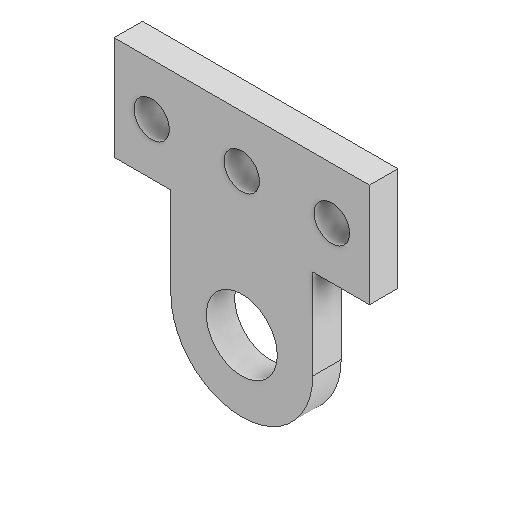
# Autodesk Inventor part: Suporte Coletor - Intake
Saved by Autodesk Inventor 2025.3 (Build 293356000, 356)
## iProperties
Created: 2026-05-13
Part Number: Suporte Coletor - Intake
Material: Genérico
Document SubType Name: Modeling
Designer: djair.oliveira
Density: 1 g/cm^3
Appearance: Padrão
Author: djair.oliveira
Autodesk Inventor part; units mm, degrees
ref_plane "YZ Plane" through (0, 0, 0) normal (1, 0, 0) x (0, 1, 0)
ref_plane "XZ Plane" through (0, 0, 0) normal (0, 1, 0) x (-1, 0, 0)
ref_plane "XY Plane" through (0, 0, 0) normal (0, 0, 1) x (1, 0, 0)
sketch "Esboço1" plane through (0, 0, 0) normal (0, 0, 1) x (1, 0, 0)
  circle A0 centre (0, 0) radius 5
  line L0 (0, 0) -> (0, 22.7) construction
  line L1 (-10, 0) -> (-10, 22.7)
  line L2 (10, 22.7) -> (10, 0)
  arc A1 (-10, 0) -> (10, 0) centre (0, 0) ccw
  arc A2 (10, 22.7) -> (-10, 22.7) centre (0, 22.7) ccw
  line L3 (-25.4, 12.7) -> (25.4, 12.7)
  line L4 (25.4, 12.7) -> (25.4, 32.7)
  line L5 (25.4, 32.7) -> (-25.4, 32.7)
  line L6 (-25.4, 32.7) -> (-25.4, 12.7)
  line L7 (-25.4, 12.7) -> (25.4, 32.7) construction
  line L8 (25.4, 12.7) -> (-25.4, 32.7) construction
  circle A3 centre (0, 20) radius 2.5
  line L9 (25.4, 12.7) -> (-25.4, 12.7)
  line L10 (-25.4, 12.7) -> (-25.4, 27.3)
  line L11 (-25.4, 27.3) -> (25.4, 27.3)
  line L12 (25.4, 27.3) -> (25.4, 12.7)
  line L13 (25.4, 12.7) -> (-25.4, 27.3) construction
  line L14 (-25.4, 12.7) -> (25.4, 27.3) construction
  circle A4 centre (12.7, 20) radius 2.5
  circle A5 centre (-12.7, 20) radius 2.5
  line L15 (18, 12.7) -> (-18, 12.7)
  line L16 (-18, 12.7) -> (-18, 27.3)
  line L17 (-18, 27.3) -> (18, 27.3)
  line L18 (18, 27.3) -> (18, 12.7)
  line L19 (18, 12.7) -> (-18, 27.3) construction
  line L20 (-18, 12.7) -> (18, 27.3) construction
  point P0 (0, 11.35)
  point P1 (25.4, 22.7)
  point P2 (-10, 12.7)
  point P3 (10, 12.7)
  dimension "d0" = 10
  dimension "d1" = 5
  dimension "d2" = 25.4
  dimension "d3" = 5
  dimension "d4" = 12.7
  dimension "d5" = 7.3
  dimension "d6" = 20
  dimension "d9" = 12.7
  dimension "d14" = 18
  constraints: 44 end point, 8 midpoint, 7 parallel, 6 centre point, 5 tangent, 4 horizontal, 4 point on circle, 3 perpendicular, 2 point on line, 1 coincident, 1 collinear, 1 vertical, 4 other
  measures "d0" diameter of A0
  measures "d1" radial gap between concentric circles of A0 A1
  measures "d2" distance of L0.end point (25.4, 22.7)
  measures "d3" diameter of A3
  measures "d4" distance from line of L5 A3.centre
  measures "d5" distance from line of L11 A3.centre
  measures "d6" distance of A3.centre point (0, 0)
  measures "d9" distance of A3.centre A4.centre
  measures "d14" distance from line of A3.centre L16
extrude "Extrusão1" add sketch "Esboço1" along normal blind 4 contours L1 L3 L2 A1 | L3 L16 L11 A2 L1 | L1 A2 L11 L2 L3 | L2 A2 L11 L18 L3
